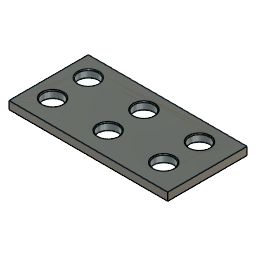
Rectangular Feature Demo Using Holes (Autodesk Fusion 360 design; units mm, degrees)
part number: 2026-06-14-15-17-23-435
Autodesk Fusion 360 part; units mm, degrees
sketch "Sketch1" plane through (0, 0, 0) normal (0, 0, 1) x (1, 0, 0)
  line L0 (100, 50) -> (-100, 50)
  line L1 (-100, 50) -> (-100, -50)
  line L2 (-100, -50) -> (100, -50)
  line L3 (100, -50) -> (100, 50)
  line L4 (100, 50) -> (-100, -50) construction
  line L5 (-100, 50) -> (100, -50) construction
  dimension "d1" = 200
  dimension "d2" = 100
  constraint horizontal L0
  constraint perpendicular L0 L1
  constraint parallel L0 L2
  constraint parallel L1 L3
  constraint coincident L4 origin
  constraint coincident L5 origin
  measures "d1" distance of L1.end L2.end
  measures "d2" distance of L0.end L1.end
extrude "Extrude1" add sketch "Sketch1" along normal blind 10
sketch "Sketch2" plane through (0, 0, 10) normal (0, 0, 1) x (-1, 0, 0)
  line L0 (-100, 50) -> (-100, -50)
  line L1 (-100, -50) -> (100, -50)
  line L2 (100, -50) -> (100, 50)
  line L3 (100, 50) -> (-100, 50)
  circle A0 centre (75, -25) radius 12.5
  dimension "d5" = 25
  dimension "d6" = 25
  dimension "d7" = 25
  measures "d5" diameter of A0
  measures "d6" distance of L1 A0.centre
  measures "d7" distance of L2 A0.centre
extrude "Extrude2" cut sketch "Sketch2" against normal blind 70 contours A0
fillet "Fillet1" radius 1 2 edges at (-63.3459, 20.4798, 10) (-63.3459, 29.5202, 0)
sketch "Sketch3" plane through (0, 0, 10) normal (0, 0, 1) x (-1, 0, 0)
  line L0 (-100, 50) -> (-100, -50)
  line L1 (-100, -50) -> (100, -50)
  line L2 (100, -50) -> (100, 50)
  line L3 (100, 50) -> (-100, 50)
  circle A0 centre (75, -25) radius 13.5
pattern_linear "R-Pattern1" count 3 spacing 70 along (1, 0, 0) count 2 spacing 45 along (0, -1, 0) of "Extrude2", "Fillet1"
